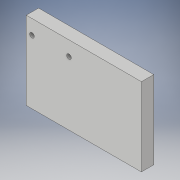
# Autodesk Inventor part: kermit bumper (small 4)
Saved by Autodesk Inventor 2018.2 (Build 222227000, 227)
## iProperties
Created: 2018-02-15
Part Number: kermit bumper (small 4)
Material: Generic
Document SubType Name: Modeling
Designer: kalra.rohan
Density: 1 g/cm^3
Appearance: Default
Author: kalra.rohan
Autodesk Inventor part; units mm, degrees
ref_plane "YZ Plane" through (0, 0, 0) normal (1, 0, 0) x (0, 1, 0)
ref_plane "XZ Plane" through (0, 0, 0) normal (0, 1, 0) x (-1, 0, 0)
ref_plane "XY Plane" through (0, 0, 0) normal (0, 0, 1) x (1, 0, 0)
sketch "Sketch1" plane through (0, 0, 0) normal (0, 0, 1) x (1, 0, 0)
  line L0 (0, 0) -> (177.8, 0)
  line L1 (177.8, 0) -> (177.8, -120.65)
  line L2 (177.8, -120.65) -> (0, -120.65)
  line L3 (0, -120.65) -> (0, 0)
  circle A0 centre (8.89, -22.352) radius 3.556
  circle A1 centre (66.04, -22.352) radius 3.556
  dimension "d0" = 177.8
  dimension "d1" = 120.65
  dimension "d2" = 7.112
  dimension "d3" = 8.89
  dimension "d4" = 98.298
  dimension "d5" = 7.112
  dimension "d6" = 98.298
  dimension "d7" = 57.15
  constraints: 8 end point, 2 centre point, 2 parallel, 1 horizontal, 1 perpendicular
  measures "d0" distance between parallel lines of L1 L3
  measures "d1" distance between parallel lines of L0 L2
  measures "d2" diameter of A0
  measures "d3" distance from line of A0.centre L3
  measures "d4" distance from line of A0.centre L2
  measures "d5" diameter of A1
  measures "d6" distance from line of A1.centre L2
  measures "d7" distance of A1.centre A0.centre
extrude "Extrusion1" add sketch "Sketch1" against normal blind 19.05
body "Solid1"
